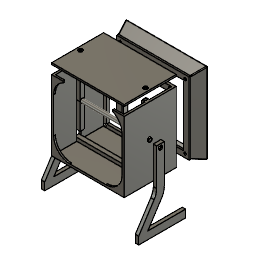
solder_fume_extractor (Autodesk Fusion 360 design; units mm, degrees)
part number: 2026-05-10-15-13-14-628
Autodesk Fusion 360 part; units mm, degrees
sketch "Sketch1" plane through (0, 0, 0) normal (0, 0, 1) x (1, 0, 0)
  line L0 (0, 0) -> (80, 0)
  line L1 (80, 0) -> (80, 80)
  line L2 (80, 80) -> (0, 80)
  line L3 (0, 80) -> (0, 0)
  line L4 (82.5, -2.5) -> (-2.5, -2.5)
  line L5 (-2.5, -2.5) -> (-2.5, 80)
  line L6 (-2.5, 80) -> (82.5, 80)
  line L7 (82.5, 80) -> (82.5, -2.5)
  line L8 (82.5, -2.5) -> (-2.5, 80) construction
  line L9 (-2.5, -2.5) -> (82.5, 80) construction
  point P0 (40, 38.75)
  dimension "d1" = 80
  dimension "d2" = 80
  dimension "d3" = 82.5
  dimension "d4" = 85
  dimension "d5" = 2.5
  constraint horizontal L0
  constraint vertical L1
  constraint horizontal L2
  constraint vertical L3
  constraint coincident L0.start L3.end
  constraint horizontal L4
  constraint perpendicular L4 L5
  constraint parallel L4 L6
  constraint parallel L5 L7
  constraint coincident L8 P0
  constraint coincident L9 P0
  measures "d1" distance of L0.start L0.end
  measures "d2" distance of L0.start L2.end
  measures "d3" distance of L4.end L5.end
  measures "d4" distance of L5.end L6.end
  measures "d5" distance of L3 L5
extrude "Extrude1" add sketch "Sketch1" along normal blind 26 contours L0 L1 L3 L4 L5 L6 L7 makes body 1
sketch "Sketch12" plane through (0, 0, 0) normal (0, 0, -1) x (-1, 0, 0)
  line L0 (-80, 80) -> (-82.5, 80)
  line L1 (-82.5, 80) -> (-82.5, -2.5)
  line L2 (-82.5, -2.5) -> (2.5, -2.5)
  line L3 (2.5, -2.5) -> (2.5, 80)
  line L4 (2.5, 80) -> (0, 80)
  line L5 (0, 80) -> (0, 0)
  line L6 (0, 0) -> (-80, 0)
  line L7 (-80, 0) -> (-80, 80)
  line L8 (-76, 4) -> (-4, 4)
  line L9 (-4, 4) -> (-4, 73.5)
  line L10 (-4, 73.5) -> (-76, 73.5)
  line L11 (-76, 73.5) -> (-76, 4)
  line L12 (0, 80) -> (-80, 80)
  line L13 (-80, 80) -> (-80, 0)
  line L14 (-80, 0) -> (0, 0)
  line L15 (0, 0) -> (0, 80)
  dimension "d34" = 6.5
  dimension "d35" = 4
  dimension "d36" = 4
  dimension "d37" = 4
  constraint horizontal L8
  constraint vertical L9
  constraint horizontal L10
  constraint vertical L11
  constraint horizontal L12
  constraint vertical L13
  constraint horizontal L14
  constraint vertical L15
  constraint coincident L6.end L7.start
  constraint coincident L4.end L5.start
  measures "d34" distance of L10 L12
  measures "d35" distance of L11 L13
  measures "d36" distance of L8 L14
  measures "d37" distance of L9 L15
extrude "Extrude12" add sketch "Sketch12" along normal blind 3 bodies 1
sketch "Sketch14" plane through (0, 0, 0) normal (0, 0, 1) x (1, 0, 0)
  line L0 (80, 0) -> (80, 80)
  line L1 (80, 80) -> (0, 80)
  line L2 (0, 80) -> (0, 0)
  line L3 (0, 0) -> (80, 0)
  line L4 (76, 73.5) -> (76, 4)
  line L5 (76, 4) -> (4, 4)
  line L6 (4, 4) -> (4, 73.5)
  line L7 (4, 73.5) -> (76, 73.5)
  circle A0 centre (78, 77.5) radius 1.5
  circle A1 centre (2, 77.5) radius 1.5
  circle A2 centre (2, 2) radius 1.5
  circle A3 centre (78, 2) radius 1.5
  dimension "d38" = 3
  dimension "d39" = 2
  dimension "d40" = 2.5
  dimension "d41" = 3
  dimension "d42" = 2.5
  dimension "d43" = 2
  dimension "d44" = 3
  dimension "d45" = 2
  dimension "d46" = 2
  dimension "d47" = 3
  dimension "d48" = 2
  dimension "d49" = 2
  measures "d38" diameter of A0
  measures "d39" distance of L0 A0.centre
  measures "d40" distance of L1 A0.centre
  measures "d41" diameter of A1
  measures "d42" distance of L1 A1.centre
  measures "d43" distance of L2 A1.centre
  measures "d44" diameter of A2
  measures "d45" distance of L2 A2.centre
  measures "d46" distance of L3 A2.centre
  measures "d47" diameter of A3
  measures "d48" distance of L0 A3.centre
  measures "d49" distance of L3 A3.centre
extrude "Extrude13" cut sketch "Sketch14" against normal blind 3 contours A0 | A1 | A2 | A3 bodies 1
sketch "Sketch17" plane through (0, 0, -3) normal (0, 0, -1) x (-1, 0, 0)
  line L0 (-82.5, 80) -> (-82.5, -2.5)
  line L1 (-82.5, -2.5) -> (2.5, -2.5)
  line L2 (2.5, -2.5) -> (2.5, 80)
  line L3 (-76, 4) -> (-76, 73.5)
  line L4 (-76, 73.5) -> (-4, 73.5)
  line L5 (-4, 73.5) -> (-4, 4)
  line L6 (-4, 4) -> (-76, 4)
  circle A0 centre (-2, 77.5) radius 1.5
  circle A1 centre (-78, 77.5) radius 1.5
  circle A2 centre (-2, 2) radius 1.5
  circle A3 centre (-78, 2) radius 1.5
  line L7 (-82.5, 82) -> (2.5, 82)
  line L8 (2.5, 80) -> (2.5, -2.5)
  line L9 (2.5, -2.5) -> (-82.5, -2.5)
  line L10 (-82.5, -2.5) -> (-82.5, 82)
  line L11 (2.5, 80) -> (2.5, 82)
extrude "Extrude15" add sketch "Sketch17" along normal blind 2 separate body contours L0 L1 L2 L7 L8 L9 L10 L11 | L3 L4 L5 L6 | A0 | A1 | A2 | A3 makes body 2
extrude "Extrude16" add 1 faces at (54.1667, 25, -5) along direction (0, 0, -1) blind 15 draft 20 on bodies 2 bodies 2
shell "Shell1" thickness 2 removed faces 1 at (55.9865, 55.6532, -20) on bodies 2
sketch "Sketch18" plane through (0, 0, -5) normal (0, 0, -1) x (-1, 0, 0)
  line L0 (-80.5, -0.5) -> (0.5, -0.5)
  line L1 (0.5, -0.5) -> (0.5, 80)
  line L2 (0.5, 80) -> (-80.5, 80)
  line L3 (-80.5, 80) -> (-80.5, -0.5)
  circle A0 centre (-78, 77.5) radius 1.5
  circle A1 centre (-2, 77.5) radius 1.5
  circle A2 centre (-78, 2) radius 1.5
  circle A3 centre (-2, 2) radius 1.5
  line L4 (-76, 75.5) -> (-4, 75.5)
  line L5 (-4, 75.5) -> (-4, 4)
  line L6 (-4, 4) -> (-76, 4)
  line L7 (-76, 4) -> (-76, 75.5)
  dimension "d59" = 3
  dimension "d60" = 2.5
  dimension "d61" = 2.5
  dimension "d62" = 3
  dimension "d63" = 2.5
  dimension "d64" = 2.5
  dimension "d65" = 3
  dimension "d66" = 2.5
  dimension "d67" = 2.5
  dimension "d68" = 3
  dimension "d69" = 2.5
  dimension "d70" = 2.5
  dimension "d71" = 4.5
  dimension "d72" = 4.5
  dimension "d73" = 4.5
  dimension "d74" = 4.5
  constraint horizontal L4
  constraint vertical L5
  constraint horizontal L6
  constraint vertical L7
  measures "d59" diameter of A0
  measures "d60" distance of L2 A0.centre
  measures "d61" distance of L3 A0.centre
  measures "d62" diameter of A1
  measures "d63" distance of L2 A1.centre
  measures "d64" distance of L1 A1.centre
  measures "d65" diameter of A2
  measures "d66" distance of L0 A2.centre
  measures "d67" distance of L3 A2.centre
  measures "d68" diameter of A3
  measures "d69" distance of L0 A3.centre
  measures "d70" distance of L1 A3.centre
  measures "d71" distance of L0 L6
  measures "d72" distance of L3 L7
  measures "d73" distance of L2 L4
  measures "d74" distance of L1 L5
extrude "Extrude17" cut sketch "Sketch18" against normal blind 2 contours A0 | A1 | A2 | A3 | L4 L5 L6 L7 bodies 2
move_body "Move1" bodies 2 to x (1, 0, 0) y (0, 1, 0) z (0, 0, 1) at (0, 0, -15)
sketch "Sketch20" plane through (0, 80, 0) normal (0, 1, 0) x (-1, 0, 0)
  line L0 (-80, 0) -> (-80, 26)
  line L1 (0, 26) -> (0, 0)
  line L2 (0, 0) -> (-80, 0)
  line L3 (-82.5, 26) -> (-82.5, -3)
  line L4 (-82.5, -3) -> (2.5, -3)
  line L5 (2.5, -3) -> (2.5, 26)
  line L6 (2.5, -3) -> (-82.5, -3)
  line L7 (-82.5, -3) -> (-82.5, 37)
  line L8 (-82.5, 37) -> (2.5, 37)
  line L9 (2.5, 37) -> (2.5, -3)
  line L10 (-80, 26) -> (-82.5, 26)
  line L11 (2.5, 26) -> (0, 26)
  dimension "d78" = 40
  constraint horizontal L6
  constraint vertical L7
  constraint horizontal L8
  constraint coincident L4.end L5.start
  measures "d78" distance of L4.end L8.end
sketch "Sketch22" plane through (0, 0, 26) normal (0, 0, 1) x (1, 0, 0)
  line L0 (82.5, 80) -> (80, 80)
  line L1 (80, 80) -> (80, 0)
  line L2 (80, 0) -> (0, 0)
  line L3 (0, 0) -> (0, 80)
  line L4 (0, 80) -> (-2.5, 80)
  line L5 (-2.5, 80) -> (-2.5, -2.5)
  line L6 (-2.5, -2.5) -> (82.5, -2.5)
  line L7 (82.5, -2.5) -> (82.5, 80)
  line L8 (76, 4) -> (4, 4)
  line L9 (4, 4) -> (4, 80)
  line L10 (4, 80) -> (76, 80)
  line L11 (76, 80) -> (76, 4)
  line L12 (-2.5, 80) -> (80, 80)
  line L13 (80, 80) -> (80, 0)
  line L14 (80, 0) -> (-2.5, 0)
  line L15 (-2.5, 0) -> (-2.5, 80)
  constraint horizontal L8
  constraint vertical L9
  constraint horizontal L10
  constraint vertical L11
  constraint horizontal L12
  constraint vertical L13
  constraint horizontal L14
  constraint vertical L15
  constraint coincident L1.end L2.start
  constraint coincident L4.end L5.start
extrude "Extrude19" add sketch "Sketch22" along normal blind 5 contours L0 L1 L2 L5 L6 L7 L13 L14 | L1 L2 L3 L8 L9 L11 L12 L13 L14 | L3 L4 L5 L12 L14 L15 bodies 1
sketch "Sketch23" plane through (0, 0, 31) normal (0, 0, 1) x (1, 0, 0)
  line L0 (-2.5, -2.5) -> (82.5, -2.5)
  line L1 (82.5, -2.5) -> (82.5, 80)
  line L2 (76, 80) -> (76, 4)
  line L3 (76, 4) -> (4, 4)
  line L4 (4, 4) -> (4, 80)
  line L5 (-2.5, 80) -> (-2.5, -2.5)
  line L6 (0, 0) -> (80, 0)
  line L7 (80, 0) -> (80, 80)
  line L8 (80, 80) -> (0, 80)
  line L9 (0, 80) -> (0, 0)
  line L10 (82.5, -2.5) -> (-2.5, -2.5)
  line L11 (-2.5, -2.5) -> (-2.5, 80)
  line L12 (-2.5, 80) -> (82.5, 80)
  line L13 (82.5, 80) -> (82.5, -2.5)
  line L14 (82.5, 80) -> (76, 80)
  line L15 (4, 80) -> (-2.5, 80)
  constraint horizontal L6
  constraint vertical L7
  constraint horizontal L8
  constraint vertical L9
  constraint coincident L6.start L9.end
  constraint horizontal L10
  constraint vertical L11
  constraint horizontal L12
  constraint vertical L13
  constraint coincident L5.start L11.end
  constraint coincident L0.end L1.start
extrude "Extrude20" add sketch "Sketch23" along normal blind 25 contours L0 L1 L5 L6 L7 L9 L10 L11 L12 L13 L14 L15 bodies 1
sketch "Sketch29" plane through (0, 0, 56) normal (0, 0, 1) x (1, 0, 0)
  line L0 (82.5, 80) -> (80, 80)
  line L1 (80, 80) -> (80, 0)
  line L2 (80, 0) -> (0, 0)
  line L3 (0, 0) -> (0, 80)
  line L4 (0, 80) -> (-2.5, 80)
  line L5 (-2.5, 80) -> (-2.5, -2.5)
  line L6 (-2.5, -2.5) -> (82.5, -2.5)
  line L7 (82.5, -2.5) -> (82.5, 80)
  line L8 (19, 80) -> (18, 80)
  line L9 (0, 62) -> (0, 61)
  line L10 (61, 80) -> (62, 80)
  line L11 (80, 62) -> (80, 61)
  line L12 (61, 0) -> (62, 0)
  line L13 (80, 18) -> (80, 19)
  line L14 (19, 0) -> (18, 0)
  line L15 (0, 18) -> (0, 19)
  arc A0 (0, 19) -> (19, 0) centre (19, 19) ccw
  line L16 (18, 0) -> (0, 0)
  line L17 (0, 0) -> (0, 18)
  arc A1 (61, 0) -> (80, 19) centre (61, 19) ccw
  line L18 (62, 0) -> (80, 0)
  line L19 (80, 0) -> (80, 18)
  arc A2 (80, 61) -> (61, 80) centre (61, 61) ccw
  line L20 (61, 80) -> (80, 80)
  line L21 (80, 80) -> (80, 61)
  arc A3 (19, 80) -> (0, 61) centre (19, 61) ccw
  line L22 (19, 80) -> (0, 80)
  line L23 (0, 80) -> (0, 61)
  line L24 (11, 80) -> (11, 78.2337)
  line L25 (69, 80) -> (69, 78.2337)
  dimension "d234" = 19
  dimension "d235" = 19
  dimension "d236" = 19
  dimension "d237" = 19
  dimension "d241" = 2.5
  dimension "d242" = 2.5
  dimension "d243" = 2.5
  dimension "d244" = 2.5
  dimension "d245" = 2.5
  dimension "d246" = 2.5
  constraint horizontal L8
  constraint vertical L9
  constraint horizontal L10
  constraint vertical L11
  constraint horizontal L12
  constraint vertical L13
  constraint horizontal L14
  constraint vertical L15
  constraint tangent L14 A0
  constraint tangent L15 A0
  constraint horizontal L16
  constraint vertical L17
  constraint tangent L12 A1
  constraint tangent L13 A1
  constraint horizontal L18
  constraint vertical L19
  constraint tangent L11 A2
  constraint tangent L10 A2
  constraint horizontal L20
  constraint vertical L21
  constraint tangent L8 A3
  constraint tangent L9 A3
  constraint horizontal L22
  constraint vertical L23
  constraint coincident L22 L24.start
  constraint coincident A3 L24.end
  constraint perpendicular L22 L24
  constraint coincident L20 L25.start
  constraint coincident A2 L25.end
  constraint perpendicular L20 L25
  measures "d234" radius of A0
  measures "d235" radius of A1
  measures "d236" radius of A2
  measures "d237" radius of A3
  measures "d241" distance of L7 L21
  measures "d242" distance of L7 L19
  measures "d243" distance of L5 L17
  measures "d244" distance of L6 L16
  measures "d245" distance of L6 L18
  measures "d246" distance of L5 L23
sketch "Sketch30" plane through (0, 80, 0) normal (0, 1, 0) x (-1, 0, 0)
  line L0 (-80, 0) -> (-80, 26)
  line L1 (-80, 26) -> (-76, 26)
  line L2 (-76, 26) -> (-76, 31)
  line L3 (-76, 31) -> (-80, 31)
  line L4 (-80, 31) -> (-80, 56)
  line L5 (-82.5, 56) -> (-82.5, -3)
  line L6 (-82.5, -3) -> (2.5, -3)
  line L7 (2.5, -3) -> (2.5, 56)
  line L8 (0, 56) -> (0, 31)
  line L9 (0, 31) -> (-4, 31)
  line L10 (-4, 31) -> (-4, 26)
  line L11 (-4, 26) -> (0, 26)
  line L12 (0, 26) -> (0, 0)
  line L13 (0, 0) -> (-80, 0)
  line L14 (2.5, -3) -> (-82.5, -3)
  line L15 (-82.5, -3) -> (-82.5, 58)
  line L16 (-82.5, 58) -> (2.5, 58)
  line L17 (2.5, 58) -> (2.5, -3)
  circle A0 centre (-2, 28.5) radius 1.5
  circle A1 centre (-78, 28.5) radius 1.5
  line L18 (-80, 56) -> (-82.5, 56)
  line L19 (2.5, 56) -> (0, 56)
  dimension "d115" = 61
  dimension "d116" = 85
  dimension "d117" = 3
  dimension "d118" = 2
  dimension "d119" = 2.5
  dimension "d120" = 3
  dimension "d121" = 2.5
  dimension "d122" = 2
  constraint horizontal L14
  constraint vertical L15
  constraint horizontal L16
  constraint vertical L17
  constraint coincident L6.end L7.start
  measures "d115" distance of L6.end L16.end
  measures "d116" distance of L6.end L5.end
  measures "d117" diameter of A0
  measures "d118" distance of L10 A0.centre
  measures "d119" distance of L11 A0.centre
  measures "d120" diameter of A1
  measures "d121" distance of L1 A1.centre
  measures "d122" distance of L2 A1.centre
extrude "Extrude26" add sketch "Sketch30" along normal blind 2 separate body makes body 3
move_body "Move2" bodies 3 to x (1, 0, 0) y (0, 1, 0) z (0, 0, 1) at (0, 10, 0)
sketch "Sketch31" plane through (0, 80, 0) normal (0, 1, 0) x (-1, 0, 0)
  line L0 (-80, 0) -> (-80, 26)
  line L1 (-80, 26) -> (-76, 26)
  line L2 (-76, 26) -> (-76, 31)
  line L3 (-76, 31) -> (-80, 31)
  line L4 (-80, 31) -> (-80, 56)
  line L5 (-82.5, 56) -> (-82.5, -3)
  line L6 (-82.5, -3) -> (2.5, -3)
  line L7 (2.5, -3) -> (2.5, 56)
  line L8 (0, 56) -> (0, 31)
  line L9 (0, 31) -> (-4, 31)
  line L10 (-4, 31) -> (-4, 26)
  line L11 (-4, 26) -> (0, 26)
  line L12 (0, 26) -> (0, 0)
  line L13 (0, 0) -> (-80, 0)
  circle A0 centre (-2, 28.5) radius 1.5
  circle A1 centre (-78, 28.5) radius 1.5
  line L14 (-80, 56) -> (-82.5, 56)
  line L15 (2.5, 56) -> (0, 56)
  dimension "d125" = 3
  dimension "d126" = 2
  dimension "d127" = 2.5
  dimension "d128" = 3
  dimension "d129" = 2
  dimension "d130" = 2.5
  measures "d125" diameter of A0
  measures "d126" distance of L10 A0.centre
  measures "d127" distance of L11 A0.centre
  measures "d128" diameter of A1
  measures "d129" distance of L2 A1.centre
  measures "d130" distance of L1 A1.centre
extrude "Extrude27" cut sketch "Sketch31" against normal blind 3 contours A0 | A1 bodies 1
sketch "Sketch33" plane through (76, 0, 0) normal (-1, 0, 0) x (0, 0, 1)
  line L0 (26, 80) -> (26, 4)
  line L1 (26, 4) -> (31, 4)
  line L2 (31, 4) -> (31, 80)
  line L3 (31, 80) -> (26, 80)
  circle A0 centre (28.5, 42) radius 2.5
  dimension "d133" = 5
  dimension "d134" = 2.5
  dimension "d135" = 38
  dimension "d136" = 38
  measures "d133" diameter of A0
  measures "d134" distance of L2 A0.centre
  measures "d135" distance of L1 A0.centre
  measures "d136" distance of L3 A0.centre
extrude "Extrude28" cut sketch "Sketch33" along normal blind 80 and the other way blind 8 contours A0 bodies 1
sketch "Sketch34" plane through (-2.5, 0, 0) normal (-1, 0, 0) x (0, 0, 1)
  circle A0 centre (28.5, 42) radius 2.5
  line L0 (-3, -2.5) -> (56, -2.5)
  line L1 (56, 80) -> (-3, 80)
  line L2 (-3, 80) -> (-3, -2.5)
  circle A1 centre (28.5, 42) radius 2.4
  line L3 (56, -2.5) -> (56, 80)
  dimension "d141" = 4.8
  constraint concentric A0 A1
  measures "d141" diameter of A1
extrude "Extrude29" add sketch "Sketch34" along normal blind 1 and the other way blind 86 separate body contours A1 makes body 4
sketch "Sketch36" plane through (-3.5, 0, 0) normal (-1, 0, 0) x (0, 0, 1)
  circle A0 centre (28.5, 42) radius 2.4
  circle A1 centre (28.5, 42) radius 1.5
  dimension "d147" = 3
  constraint concentric A0 A1
  measures "d147" diameter of A1
extrude "Extrude30" cut sketch "Sketch36" against normal blind 3 contours A1 bodies 4
sketch "Sketch37" plane through (83.5, 0, 0) normal (1, 0, 0) x (0, 0, -1)
  circle A0 centre (-28.5, 42) radius 2.4
  circle A1 centre (-28.5, 42) radius 1.5
  dimension "d150" = 3
  constraint concentric A0 A1
  measures "d150" diameter of A1
extrude "Extrude31" cut sketch "Sketch37" against normal blind 3 contours A1 bodies 4
sketch "Sketch40" plane through (83.5, 0, 0) normal (1, 0, 0) x (0, 0, -1)
  circle A0 centre (-28.5, 42) radius 1.5
  circle A1 centre (-28.5, 42) radius 2.4
  line L0 (-20, 46) -> (-11, 46)
  line L1 (-11, 46) -> (-11, -2.5)
  line L2 (-11, -2.5) -> (-20, -2.5)
  line L3 (-20, -2.5) -> (-20, 46)
  line L4 (14, -35) -> (-41, -35)
  line L5 (-41, -35) -> (-41, -44)
  line L6 (-41, -44) -> (14, -44)
  line L7 (14, -44) -> (14, -35)
  line L8 (-20, -2.5) -> (-41, -35)
  line L9 (-41, -35) -> (-33.4408, -39.8844)
  line L10 (-33.4408, -39.8844) -> (-12.4408, -7.3844)
  line L11 (-12.4408, -7.3844) -> (-20, -2.5)
  line L12 (-11, -2.5) -> (-12.4408, -7.3844)
  dimension "d157" = 9
  dimension "d162" = 9
  dimension "d164" = 9
  constraint horizontal L0
  constraint vertical L1
  constraint horizontal L2
  constraint vertical L3
  constraint horizontal L4
  constraint vertical L5
  constraint horizontal L6
  constraint vertical L7
  constraint perpendicular L8 L9
  constraint parallel L8 L10
  constraint parallel L9 L11
  measures "d157" distance of L0.start L0.end
  measures "d162" distance of L4.start L6.end
  measures "d164" distance of L2.end L10.end
extrude "Extrude33" add sketch "Sketch40" along normal blind 4 separate body contours L0 L1 L2 L3 | L4 L8 L10 L11 | L2 L11 L12 | L4 L5 L6 L7 L9 L10 | L4 L9 L10 makes body 5
fillet "Fillet7" radius 0.8 8 edges at (40, 87.4596, -35) (85.2298, 84.7298, -27.5) (-5.2298, 84.7298, -27.5) (-7.9596, 39.75, -35) (87.9596, 39.75, -35) (40, -7.9596, -35) (85.2298, -5.2298, -27.5) (-5.2298, -5.2298, -27.5) on bodies 2
fillet "Fillet8" radius 0.8 4 edges at (85.8312, 39.75, -35) (40, -5.8312, -35) (40, 85.3312, -35) (-5.8312, 39.75, -35) on bodies 2
move_body "Move3" bodies 5 to x (1, 0, 0) y (0, 1, 0) z (0, 0, 1) at (10, 0, 0)
fillet "Fillet9" radius 18 2 edges at (95.5, -2.5, 11) (95.5, -7.3844, 12.4408) on bodies 5
fillet "Fillet10" radius 18 1 edges at (95.5, -2.5, 20) on bodies 5
sketch "Sketch42" plane through (4, 0, 0) normal (1, 0, 0) x (0, 0, -1)
  arc A0 (-31, 42) -> (-26, 42) centre (-28.5, 42) ccw
  line L0 (-31, 42) -> (-31, 4)
  line L1 (-31, 4) -> (-26, 4)
  line L2 (-26, 4) -> (-26, 42)
  line L3 (-31, 4) -> (-26, 4)
  line L4 (-26, 4) -> (-26, 11.9761)
  line L5 (-26, 11.9761) -> (-31, 11.9761)
  line L6 (-31, 11.9761) -> (-31, 4)
  constraint horizontal L3
  constraint vertical L4
  constraint horizontal L5
  constraint vertical L6
  constraint coincident L2 L4.end
  constraint coincident L0.end L1.start
extrude "Extrude34" cut sketch "Sketch42" against normal blind 9 contours L0 L1 L2 L3 L4 L5 L6 bodies 1
sketch "Sketch45" plane through (-2.5, 0, 0) normal (-1, 0, 0) x (0, 0, 1)
  line L0 (-3, -2.5) -> (56, -2.5)
  line L1 (56, 80) -> (-3, 80)
  line L2 (-3, 80) -> (-3, -2.5)
  circle A0 centre (28.5, 42) radius 2.5
  line L3 (17, 74) -> (26, 74)
  line L4 (26, 74) -> (26, 60)
  line L5 (26, 60) -> (17, 60)
  line L6 (17, 60) -> (17, 74)
  line L7 (31, 4) -> (26, 4)
  line L8 (26, 4) -> (26, 11.9761)
  line L9 (26, 11.9761) -> (31, 11.9761)
  line L10 (31, 11.9761) -> (31, 4)
  line L11 (56, -2.5) -> (56, 80)
  dimension "d196" = 14
  dimension "d197" = 9
  dimension "d199" = 6
  dimension "d240" = 30
  constraint horizontal L3
  constraint vertical L4
  constraint horizontal L5
  constraint vertical L6
  measures "d196" distance of L3.start L5.end
  measures "d197" distance of L3.start L3.end
  measures "d199" distance of L1 L3
  measures "d240" distance of L4 L11
extrude "Extrude36" cut sketch "Sketch45" against normal blind 7 contours L3 L4 L5 L6 bodies 1
sketch "Sketch46" plane through (97.5, 0, 0) normal (1, 0, 0) x (0, 0, -1)
  arc A0 (-13.8815, -9.6142) -> (-11, 0.1547) centre (-29, 0.1547) ccw
  line L0 (-11, 0.1547) -> (-11, 46)
  line L1 (-11, 46) -> (-20, 46)
  line L2 (-20, 46) -> (-20, 2.8094)
  arc A1 (-22.8815, -6.9595) -> (-20, 2.8094) centre (-38, 2.8094) ccw
  line L3 (-22.8815, -6.9595) -> (-41, -35)
  line L4 (-41, -35) -> (-41, -44)
  line L5 (-41, -44) -> (14, -44)
  line L6 (14, -44) -> (14, -35)
  line L7 (14, -35) -> (-30.2847, -35)
  line L8 (-30.2847, -35) -> (-13.8815, -9.6142)
  circle A2 centre (-15.5, 42) radius 2.5
extrude "Extrude37" cut sketch "Sketch46" against normal blind 1 contours A2 bodies 5
sketch "Sketch47" plane through (0, 92, 0) normal (0, 1, 0) x (-1, 0, 0)
  circle A0 centre (-2, 28.5) radius 1.5
  circle A1 centre (-78, 28.5) radius 1.5
  line L0 (2.5, 58) -> (-82.5, 58)
  line L1 (-82.5, 58) -> (-82.5, -3)
  line L2 (-82.5, -3) -> (2.5, -3)
  line L3 (2.5, -3) -> (2.5, 58)
  circle A2 centre (-2, 28.5) radius 2.5
  circle A3 centre (-78, 28.5) radius 2.5
  dimension "d205" = 5
  dimension "d206" = 5
  constraint concentric A0 A2
  constraint concentric A1 A3
  measures "d205" diameter of A2
  measures "d206" diameter of A3
extrude "Extrude38" cut sketch "Sketch47" against normal blind 1 contours A2 | A3 bodies 3
sketch "Sketch48" plane through (0, 0, -20) normal (0, 0, -1) x (-1, 0, 0)
  line L0 (0.5, -0.5) -> (0.5, 80)
  line L1 (0.5, 80) -> (-80.5, 80)
  line L2 (-80.5, 80) -> (-80.5, -0.5)
  line L3 (-80.5, -0.5) -> (0.5, -0.5)
  circle A0 centre (-2, 2) radius 1.5
  circle A1 centre (-2, 77.5) radius 1.5
  circle A2 centre (-78, 2) radius 1.5
  line L4 (-4, 75.5) -> (-4, 4)
  line L5 (-4, 4) -> (-76, 4)
  line L6 (-76, 4) -> (-76, 75.5)
  line L7 (-76, 75.5) -> (-4, 75.5)
  circle A3 centre (-78, 77.5) radius 1.5
  circle A4 centre (-2, 2) radius 2.5
  circle A5 centre (-78, 2) radius 2.5
  circle A6 centre (-78, 77.5) radius 2.5
  circle A7 centre (-2, 77.5) radius 2.5
  dimension "d209" = 5
  dimension "d210" = 5
  dimension "d211" = 5
  dimension "d212" = 5
  constraint concentric A0 A4
  constraint concentric A2 A5
  constraint concentric A3 A6
  constraint concentric A1 A7
  measures "d209" diameter of A4
  measures "d210" diameter of A5
  measures "d211" diameter of A6
  measures "d212" diameter of A7
extrude "Extrude39" cut sketch "Sketch48" against normal blind 1 contours A4 | A7 | A5 | A6 bodies 2
copy_body "CopyPasteBodies3" bodies 5 makes body 6
move_body "Move6" bodies 6 to x (1, 0, 0) y (0, 1, 0) z (0, 0, 1) at (-110, 0, 0)
extrude "Extrude40" add 1 faces at (-13.5, 41.2849, 14.7744) along direction (1, 0, 0) blind 1 on bodies 6 bodies 6
sketch "Sketch49" plane through (-16.5, 0, 0) normal (-1, 0, 0) x (0, 0, 1)
  arc A0 (11, 0.1547) -> (13.8815, -9.6142) centre (29, 0.1547) ccw
  line L0 (13.8815, -9.6142) -> (30.2847, -35)
  line L1 (30.2847, -35) -> (-14, -35)
  line L2 (-14, -35) -> (-14, -44)
  line L3 (-14, -44) -> (41, -44)
  line L4 (41, -44) -> (41, -35)
  line L5 (41, -35) -> (22.8815, -6.9595)
  arc A1 (20, 2.8094) -> (22.8815, -6.9595) centre (38, 2.8094) ccw
  line L6 (20, 2.8094) -> (20, 46)
  line L7 (20, 46) -> (11, 46)
  line L8 (11, 46) -> (11, 0.1547)
  circle A2 centre (15.5, 42) radius 2.5
  dimension "d217" = 5
  measures "d217" diameter of A2
extrude "Extrude41" cut sketch "Sketch49" against normal blind 1 contours A2 bodies 6
move_body "Move7" bodies 6 5 to x (1, 0, 0) y (0, 1, 0) z (0, 0, 1) at (0, 0, 15)
sketch "Sketch50" plane through (-15.5, 0, 0) normal (-1, 0, 0) x (0, 0, 1)
  circle A0 centre (30.5, 42) radius 2.5
  circle A1 centre (30.5, 42) radius 1.5
  dimension "d220" = 3
  constraint concentric A0 A1
  measures "d220" diameter of A1
extrude "Extrude42" cut sketch "Sketch50" against normal blind 3.5 contours A1 bodies 6
sketch "Sketch51" plane through (96.5, 0, 0) normal (1, 0, 0) x (0, 0, -1)
  circle A0 centre (-30.5, 42) radius 2.5
  circle A1 centre (-30.5, 42) radius 1.5
  dimension "d223" = 3
  constraint concentric A0 A1
  measures "d223" diameter of A1
extrude "Extrude43" cut sketch "Sketch51" against normal blind 3 contours A1 bodies 5
extrude "Extrude45" add sketch "Sketch29" along normal blind 2 contours L0 L1 L2 L3 L4 L5 L6 L7 L9 L11 L12 L13 L14 L15 L16 L17 L18 L19 L21 L23 | L1 L11 A2 L20 L21 L25 | L1 L2 L12 L13 A1 L18 L19 | L3 L9 A3 L22 L23 L24 | L2 L3 L14 L15 A0 L16 L17 bodies 1
named bodies: "Body", "Head", "Top", "Pole", "Leg_R", "Leg_L"
